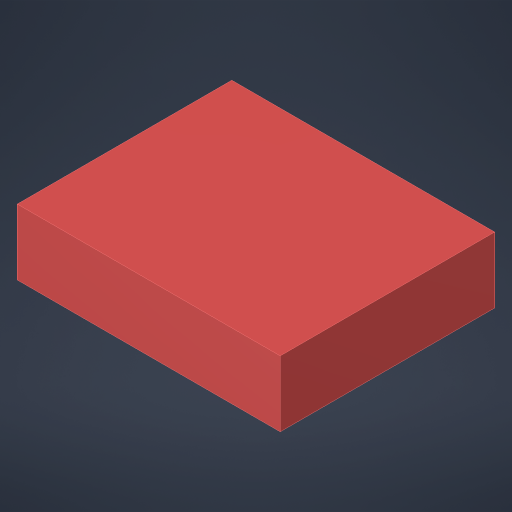
# Autodesk Inventor part: big craftsman
Saved by Autodesk Inventor 2023.4 (Build 274418000, 418)
## iProperties
Created: 2025-03-02
Part Number: big craftsman
Material: Aluminum 6061
Document SubType Name: Modeling
Designer: brand
Density: 2.7 g/cm^3
Appearance: Smooth - Red
Author: brand
Autodesk Inventor part; units mm, degrees
ref_plane "YZ Plane" through (0, 0, 0) normal (1, 0, 0) x (0, 1, 0)
ref_plane "XZ Plane" through (0, 0, 0) normal (0, 1, 0) x (-1, 0, 0)
ref_plane "XY Plane" through (0, 0, 0) normal (0, 0, 1) x (1, 0, 0)
sketch "Sketch1" plane through (0, 0, 0) normal (0, 1, 0) x (-1, 0, 0)
  line L0 (241.3, 196.85) -> (-241.3, 196.85)
  line L1 (-241.3, 196.85) -> (-241.3, -196.85)
  line L2 (-241.3, -196.85) -> (241.3, -196.85)
  line L3 (241.3, -196.85) -> (241.3, 196.85)
  line L4 (241.3, 196.85) -> (-241.3, -196.85) construction
  line L5 (-241.3, 196.85) -> (241.3, -196.85) construction
  point P0 (0, 0)
  dimension "d0" = 482.6
  dimension "d1" = 393.7
  constraints: 12 end point, 2 midpoint, 2 parallel, 1 horizontal, 1 perpendicular
  measures "d0" distance of L2.end L1.end
  measures "d1" distance of L1.end L0.end
extrude "Extrusion1" add sketch "Sketch1" along normal mid plane 120.65
body "Solid1"
